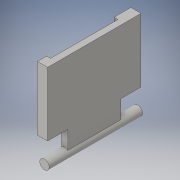
# Autodesk Inventor part: gpsDoor
Saved by Autodesk Inventor 2016 (Build 200138000, 138)
## iProperties
Created: 2016-10-13
Part Number: gpsDoor
Material: Generic
Document SubType Name: Modeling
Designer: lachesis
Density: 1 g/cm^3
Appearance: Default
Author: lachesis
Autodesk Inventor part; units mm, degrees
ref_plane "YZ Plane" through (0, 0, 0) normal (1, 0, 0) x (0, 1, 0)
ref_plane "XZ Plane" through (0, 0, 0) normal (0, 1, 0) x (-1, 0, 0)
ref_plane "XY Plane" through (0, 0, 0) normal (0, 0, 1) x (1, 0, 0)
sketch "Sketch1" plane through (0, 0, 0) normal (0, 0, 1) x (1, 0, 0)
  circle A0 centre (0, 0) radius 1.5
  dimension "d0" = 3
  constraints: 1 centre point, 1 coincident
  measures "d0" diameter of A0
extrude "Extrusion1" add sketch "Sketch1" along normal blind 30
ref_plane "Work Plane1" through (0, 0, 23.5) normal (0, 0, 1) x (1, 0, 0)
ref_plane "Work Plane2" through (0, 0, 6.5) normal (0, 0, -1) x (-1, 0, 0)
sketch "Sketch2" plane through (0, 0, 23.5) normal (0, 0, 1) x (1, 0, 0)
  circle A0 centre (0, 0) radius 1.5 projected
  line L0 (1, 0) -> (-1, 0)
  line L1 (-1, 0) -> (-1, 27.5)
  line L2 (-1, 27.5) -> (1, 27.5)
  line L3 (1, 27.5) -> (1, 0)
  dimension "d7" = 27.5
  dimension "d13" = 1
  constraints: 8 end point, 2 parallel, 1 coincident, 1 horizontal, 1 midpoint, 1 perpendicular
  measures "d7" distance from line of point (0, 0) L2
  measures "d13" distance from line of point (0, 0) L1
extrude "Extrusion2" add sketch "Sketch2" against normal up to surface (17 mm away) contours L3 L0 L1 A0 | A0 L1 L2 L3 picked at (0, 0.5)
sketch "Sketch3" plane through (1, 1.118, 23.5) normal (1, 0, 0) x (0, 0, -1)
  line L0 (17, 0) -> (17, 26.382) projected
  line L1 (0, 26.382) -> (17, 26.382) projected
  line L2 (0, 26.382) -> (0, 0) projected
  line L3 (17, 0) -> (0, 0) projected
  line L4 (0, 26.382) -> (-6.5, 26.382)
  line L5 (-6.5, 26.382) -> (-6.5, 5.882)
  line L6 (-6.5, 5.882) -> (0, 5.882)
  line L7 (0, 5.882) -> (0, 26.382)
  line L8 (17, 0) -> (17, 26.382) projected
  line L9 (17, 26.382) -> (23.5, 26.382)
  line L10 (23.5, 26.382) -> (23.5, 5.882)
  line L11 (23.5, 5.882) -> (17, 5.882)
  line L12 (17, 5.882) -> (17, 26.382)
  line L13 (23.5, -2.618) -> (23.5, 0.382) projected
  line L14 (-6.5, 0.382) -> (-6.5, -2.618) projected
  line L15 (0, 0) -> (17, 0) projected
  line L16 (17, 0) -> (17, 0) projected
  line L17 (17, 0) -> (0, 0) projected
  line L18 (0, 0) -> (0, 0) projected
  point P0 (23.5, -1.118)
  point P1 (20.25, 5.882)
  point P2 (-3.25, 5.882)
  point P3 (23.5, -1.118)
  point P4 (23.5, 16.132)
  point P5 (-6.5, 16.132)
  point P6 (-6.5, -1.118)
  dimension "d10" = 5.5
  constraints: 16 end point, 6 midpoint, 4 parallel, 2 horizontal, 2 perpendicular, 2 vertical alignment, 1 horizontal alignment
  measures "d10" distance from line of L13.end L11
extrude "Extrusion3" add sketch "Sketch3" against normal up to surface (2 mm away) contours L0 L9 L10 L11 | L6 L5 L4 L2
sketch "Sketch5" plane through (-1, 1.118, 6.5) normal (-1, 0, 0) x (0, 0, 1)
  line L0 (17, 0) -> (0, 0) projected
  line L1 (17, 0) -> (17, 5.882) projected
  line L2 (23.5, 5.882) -> (17, 5.882) projected
  line L3 (23.5, 26.382) -> (23.5, 5.882) projected
  line L4 (23.5, 26.382) -> (-6.5, 26.382) projected
  line L5 (-6.5, 5.882) -> (-6.5, 26.382) projected
  line L6 (0, 5.882) -> (-6.5, 5.882) projected
  line L7 (0, 5.882) -> (0, 0) projected
  line L8 (23.5, 5.882) -> (17, 5.882) projected
  line L9 (23.5, 26.382) -> (-6.5, 26.382) projected
  line L10 (23.5, 5.882) -> (20.5, 5.882)
  line L11 (20.5, 5.882) -> (20.5, 26.382)
  line L12 (20.5, 26.382) -> (23.5, 26.382)
  line L13 (23.5, 26.382) -> (23.5, 5.882)
  line L14 (0, 5.882) -> (-6.5, 5.882) projected
  line L15 (-6.5, 26.382) -> (-1.1, 26.382)
  line L16 (-1.1, 26.382) -> (-1.1, 5.882)
  line L17 (-1.1, 5.882) -> (-6.5, 5.882)
  line L18 (-6.5, 5.882) -> (-6.5, 26.382)
  point P0 (-6.5, -1.118)
  dimension "d16" = 3
  dimension "d17" = 5.4
  constraints: 16 end point, 4 parallel, 2 horizontal, 2 perpendicular, 2 point on line
  measures "d16" distance between parallel lines of L3 L11
  measures "d17" distance between parallel lines of L16 L5
extrude "Extrusion5" add sketch "Sketch5" along normal blind 1.26 contours L11 L4 L3 L2 | L6 L5 L4 L16
body "Solid1"
